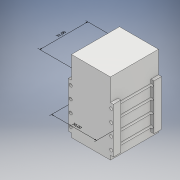
# Autodesk Inventor part: ax12
Saved by Autodesk Inventor 2018 (Build 220112000, 112)
## iProperties
Created: 2017-11-23
Part Number: ax12
Material: ABS Plastic
Document SubType Name: Modeling
Designer: Biscuit
Density: 1.06 g/cm^3
Appearance: Smooth - White
Author: Biscuit
Autodesk Inventor part; units mm, degrees
ref_plane "YZ Plane" through (0, 0, 0) normal (1, 0, 0) x (0, 1, 0)
ref_plane "XZ Plane" through (0, 0, 0) normal (0, 1, 0) x (-1, 0, 0)
ref_plane "XY Plane" through (0, 0, 0) normal (0, 0, 1) x (1, 0, 0)
sketch "Sketch1" plane through (0, 0, 0) normal (0, 1, 0) x (-1, 0, 0)
  line L0 (0, 0) -> (26, 0)
  line L1 (26, 0) -> (26, -48)
  line L2 (26, -48) -> (0, -48)
  line L3 (0, -48) -> (0, 0)
  dimension "d0" = 26
  dimension "d1" = 48
  constraints: 8 end point, 2 parallel, 1 horizontal, 1 perpendicular
  measures "d0" distance of L0.start L0.end
  measures "d1" distance of L0.end L1.end
extrude "Extrusion1" add sketch "Sketch1" along normal blind 32
sketch "Sketch2" plane through (0, 32, 0) normal (0, 1, 0) x (1, 0, 0)
  circle A0 centre (-13, 11.5) radius 3.5
  line L0 (0, 0) -> (-26, 0) projected
  line L1 (0, 0) -> (0, 48) projected
  dimension "d4" = 7
  dimension "d5" = 11.5
  dimension "d6" = 26
  dimension "d7" = 13
  constraints: 1 centre point
  measures "d4" diameter of A0
  measures "d5" distance from line of L0 A0.centre
  measures "d6" distance of L0.start L0.end
  measures "d7" distance from line of L1 A0.centre
extrude "Extrusion2" cut sketch "Sketch2" against normal blind 10
sketch "Sketch3" plane through (0, 0, 0) normal (1, 0, 0) x (0, 0, -1)
  line L0 (0, 32) -> (48, 32) projected
  line L1 (14.75, 32) -> (45.25, 32)
  line L2 (45.25, 32) -> (45.25, 27)
  line L3 (45.25, 27) -> (14.75, 27)
  line L4 (14.75, 27) -> (14.75, 32)
  line L5 (48, 0) -> (0, 0) projected
  line L6 (45.25, 0) -> (14.75, 0)
  line L7 (14.75, 0) -> (14.75, 5)
  line L8 (14.75, 5) -> (45.25, 5)
  line L9 (45.25, 5) -> (45.25, 0)
  line L10 (0, 0) -> (0, 32) projected
  line L11 (48, 0) -> (48, 32) projected
  dimension "d10" = 5
  dimension "d11" = 5
  dimension "d12" = 30.5
  dimension "d13" = 30.5
  dimension "d52" = 14.75
  constraints: 16 end point, 4 parallel, 4 point on line, 2 horizontal, 2 perpendicular
  measures "d10" distance of L6.end L7.end
  measures "d11" distance of L3.end L1.start
  measures "d12" distance of L2.end L3.end
  measures "d13" distance of L7.end L8.end
  measures "d52" distance between parallel lines of L10 L4
extrude "Extrusion3" add sketch "Sketch3" along normal blind 2 contours L0 L2 L3 L4 | L7 L8 L9 L5
sketch "Sketch4" plane through (-26, 0, -48) normal (-1, 0, 0) x (0, 0, 1)
  line L0 (2.75, 27) -> (2.75, 32) projected
  line L1 (2.75, 32) -> (33.25, 32) projected
  line L2 (33.25, 32) -> (33.25, 27) projected
  line L3 (33.25, 27) -> (2.75, 27) projected
  line L4 (2.75, 27) -> (2.75, 32) projected
  line L5 (33.25, 0) -> (2.75, 0) projected
  line L6 (2.75, 0) -> (2.75, 5) projected
  line L7 (2.75, 5) -> (33.25, 5) projected
  line L8 (33.25, 5) -> (33.25, 0) projected
  point P0 (48, 0)
extrude "Extrusion4" add sketch "Sketch4" along normal blind 2
sketch "Sketch5" plane through (0, 32, 0) normal (0, 1, 0) x (1, 0, 0)
  circle A0 centre (0.5, 42) radius 1
  line L0 (0, 45.25) -> (2, 45.25) projected
  line L1 (2, 45.25) -> (2, 14.75) projected
  circle A1 centre (-13, 11.5) radius 3.5 projected
  line L2 (-26, 0) -> (0, 0) projected
  line L3 (0, 0) -> (0, 14.75) projected
  line L4 (0, 14.75) -> (2, 14.75) projected
  line L5 (2, 45.25) -> (2, 14.75) projected
  line L6 (0, 45.25) -> (2, 45.25) projected
  line L7 (0, 48) -> (-26, 48) projected
  line L8 (-26, 48) -> (-26, 45.25) projected
  line L9 (-26, 45.25) -> (-28, 45.25) projected
  line L10 (-28, 14.75) -> (-28, 45.25) projected
  line L11 (-26, 14.75) -> (-28, 14.75) projected
  circle A2 centre (0.5, 34) radius 1
  circle A3 centre (0.5, 26) radius 1
  circle A4 centre (0.5, 18) radius 1
  circle A5 centre (-26.5, 42) radius 1
  circle A6 centre (-26.5, 34) radius 1
  circle A7 centre (-26.5, 26) radius 1
  circle A8 centre (-26.5, 18) radius 1
  line L12 (0, 45.25) -> (0, 48) projected
  line L13 (-26, 14.75) -> (-26, 0) projected
  point P0 (0, 48.5)
  dimension "d20" = 2
  dimension "d21" = 3.25
  dimension "d24" = 8
  dimension "d29" = 3.25
  dimension "d30" = 1.5
  dimension "d32" = 2
  dimension "d33" = 1.5
  dimension "d36" = 8
  dimension "d41" = 3.25
  dimension "d42" = 3.25
  constraints: 8 centre point, 2 vertical, 13 other
  measures "d20" diameter of A0
  measures "d24" distance of A0.centre A2.centre
  measures "d29" distance from line of L4 A4.centre
  measures "d30" distance from line of L1 A0.centre
  measures "d32" diameter of A5
  measures "d33" distance from line of L10 A5.centre
  measures "d36" distance of A5.centre A6.centre
  measures "d41" distance from line of L11 A8.centre
  measures "d42" distance from line of L9 A5.centre
extrude "Extrusion5" cut sketch "Sketch5" against normal through all contours A0 | A2 | A3 | A4 | A5 | A6 | A7 | A8
equation "\"d7\" = 0.5 * d6"
equation "\"d10\" = d11"
equation "\"d21\" = d29"
equation "\"d41\" = d42"
body "Solid1"
